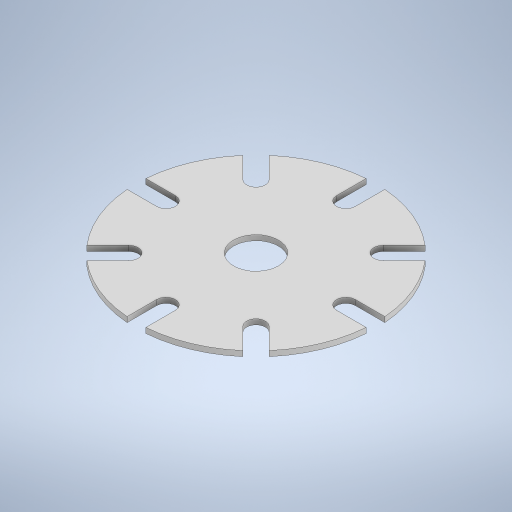
# Autodesk Inventor part: Disc
Saved by Autodesk Inventor 2023 (Build 270158000, 158)
## iProperties
Created: 2023-06-14
Part Number: Disc
Material: Generisch
Document SubType Name: Modeling
Designer: prigge
Density: 1 g/cm^3
Appearance: Vorgabe
Author: prigge
Autodesk Inventor part; units mm, degrees
ref_plane "YZ Plane" through (0, 0, 0) normal (1, 0, 0) x (0, 1, 0)
ref_plane "XZ Plane" through (0, 0, 0) normal (0, 1, 0) x (-1, 0, 0)
ref_plane "XY Plane" through (0, 0, 0) normal (0, 0, 1) x (1, 0, 0)
sketch "Skizze1" plane through (0, 0, 0) normal (0, 1, 0) x (-1, 0, 0)
  circle A0 centre (0, 0) radius 3
  circle A1 centre (0, 0) radius 16
  dimension "d0" = 6
  dimension "d1" = 32
  constraints: 2 centre point, 2 coincident
  measures "d0" diameter of A0
  measures "d1" diameter of A1
extrude "Extrusion1" add sketch "Skizze1" along normal blind 0.7
sketch "Skizze2" plane through (0, 0.7, 0) normal (0, 1, 0) x (1, 0, 0)
  circle A0 centre (0, 0) radius 16 projected
  line L0 (-15.9511, -1.25) -> (-12, -1.25)
  arc A1 (-12, -1.25) -> (-12, 1.25) centre (-12, 0) ccw
  line L1 (-12, 1.25) -> (-15.9511, 1.25)
  point P0 (-13.9755, -1.25)
  dimension "d4" = 12
  dimension "d5" = 2.5
  constraints: 4 end point, 4 point on circle, 2 horizontal, 2 tangent, 1 centre point, 1 midpoint
  measures "d4" distance of point (0, 0) A1.centre
  measures "d5" distance from line of point (-13.976, -1.25) L1
extrude "Extrusion2" cut sketch "Skizze2" against normal blind 0.7 contours L1 A1 L0 A0 picked at (-13.3315, -0.139)
pattern_circular "Runde Anordnung1" count 8 over 360 about axis through (0, -10, 0) along (0, 1, 0) of "Extrusion2"
